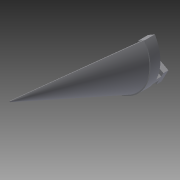
# Autodesk Inventor part: Pá 120
Saved by Autodesk Inventor 2015 (Build 190159000, 159)
## iProperties
Created: 2016-04-14
Part Number: Pá 120
Material: Generic
Document SubType Name: Modeling
Designer: Diogo Figueiredo
Density: 1 g/cm^3
Appearance: Default
Author: Diogo Figueiredo
Autodesk Inventor part; units mm, degrees
ref_plane "YZ Plane" through (0, 0, 0) normal (1, 0, 0) x (0, 1, 0)
ref_plane "XZ Plane" through (0, 0, 0) normal (0, 1, 0) x (-1, 0, 0)
ref_plane "XY Plane" through (0, 0, 0) normal (0, 0, 1) x (1, 0, 0)
sketch "Sketch1" plane through (0, 0, 0) normal (1, 0, 0) x (0, 1, 0)
  line L0 (0, 0) -> (100, 0)
  line L1 (100, 0) -> (100, -40)
  line L2 (0, 0) -> (0, -1)
  line L3 (0, -1) -> (100, -40)
  line L4 (100, -40) -> (100, -38)
  line L5 (100, -38) -> (0, 0)
  line L6 (100, -40) -> (100, -41)
  line L7 (100, -41) -> (110, -41)
  line L8 (110, -41) -> (110, -33)
  line L9 (110, -33) -> (100, -33)
  dimension "d0" = 100
  dimension "d1" = 40
  dimension "d2" = 1
  dimension "d3" = 2
  dimension "d7" = 1
  dimension "d8" = 10
  dimension "d9" = 8
  constraints: 20 end point, 3 perpendicular, 3 vertical, 2 point on line, 1 horizontal
  measures "d0" distance of L0.start L0.end
  measures "d1" distance of L0.end L1.end
  measures "d2" distance of L0.start L2.end
  measures "d3" distance of L1.end L4.end
  measures "d7" distance of L1.end L6.end
  measures "d8" distance of L6.end L7.end
  measures "d9" distance of L7.end L8.end
revolve "Revolution1" add sketch "Sketch1" angle 120 about axis through (0, 0, 0) along (0, -1, 0) contours L5 L1 L3 L2 | L1 L9 L8 L7 L6
sketch "Sketch2" plane through (0, 110, -33) normal (0, 1, 0) x (1, 0, 0)
  line L0 (32.909, -14) -> (35.507, -12.5)
  line L1 (35.507, -12.5) -> (33.913, -9.9585)
  line L2 (35.507, -12.5) -> (36.911, -15.1512)
  line L3 (36.911, -15.1512) -> (23.6549, -22.1709)
  line L4 (23.6549, -22.1709) -> (20.847, -16.8685)
  line L5 (20.847, -16.8685) -> (33.913, -9.9585)
  dimension "d11" = 3
  dimension "d12" = 3
  dimension "d13" = 15
  dimension "d14" = 6
  constraints: 12 end point, 2 perpendicular
  measures "d11" distance of L0.end L1.end
  measures "d12" distance of L0.end L2.end
  measures "d13" distance of L2.end L3.end
  measures "d14" distance of L3.end L4.end
extrude "Extrusion1" add sketch "Sketch2" along normal mid plane 20
sketch "Sketch3" plane through (23.6549, 100, -10.8291) normal (-0.8837, 0, 0.468) x (0.468, 0, 0.8837)
  line L0 (-3, 20) -> (4.5, 20)
  line L1 (4.5, 20) -> (4.5, 15)
  line L2 (4.5, 15) -> (-10.5, 15)
  line L3 (-10.5, 15) -> (-10.5, 20)
  line L4 (-10.5, 20) -> (-3, 20)
  point P0 (-1.5, -100)
  dimension "d17" = 7.5
  dimension "d18" = 5
  dimension "d19" = 15
  constraints: 10 end point, 3 perpendicular, 1 collinear, 1 horizontal, 1 point on line
  measures "d17" distance of L0.start L0.end
  measures "d18" distance of L0.end L1.end
  measures "d19" distance of L1.end L2.end
extrude "Extrusion2" add sketch "Sketch3" against normal blind 15
body "Solid1"
